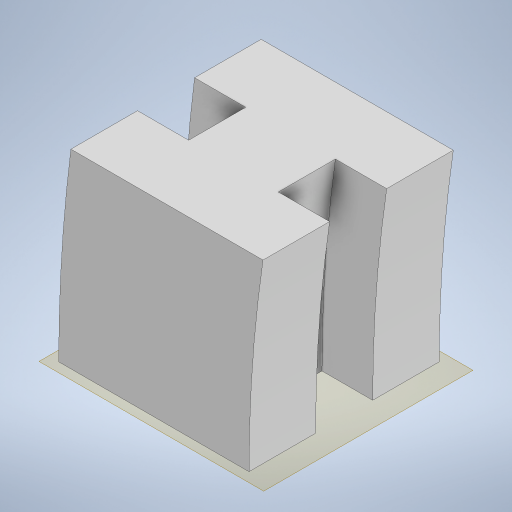
# Autodesk Inventor part: LightRail01
Saved by Autodesk Inventor 2023 (Build 270158000, 158)
## iProperties
Created: 2023-04-11
Part Number: LightRail01
Material: Generic
Document SubType Name: Modeling
Designer: ringl
Density: 1 g/cm^3
Appearance: Default
Author: ringl
Autodesk Inventor part; units mm, degrees
ref_plane "YZ Plane" through (0, 0, 0) normal (1, 0, 0) x (0, 1, 0)
ref_plane "XY Plane" through (0, 0, 0) normal (0, 0, 1) x (1, 0, 0)
sketch "Sketch1" plane through (0, 0, 0) normal (0, 0, 1) x (1, 0, 0)
  arc A0 (440, 0) -> (0, 0) centre (220, 0) ccw
  dimension "d1" = 440
  dimension "d17" = 220
  constraints: 2 point on circle, 1 centre point, 1 horizontal alignment
  measures "d1" distance of A0.end A0.start
  measures "d17" radius of A0
sketch "Sketch2" plane through (0, 0, 0) normal (0, 1, 0) x (-1, 0, 0)
  line L0 (15, 15) -> (-15, 15)
  line L1 (-15, -15) -> (15, -15)
  line L2 (15, 4.5) -> (7, 4.5)
  line L3 (7, 4.5) -> (7, -4.5)
  line L4 (7, -4.5) -> (15, -4.5)
  line L5 (-15, 4.5) -> (-7, 4.5)
  line L6 (-7, 4.5) -> (-7, -4.5)
  line L7 (-7, -4.5) -> (-15, -4.5)
  line L8 (15, -15) -> (15, -4.5)
  line L9 (15, 4.5) -> (15, 15)
  line L10 (-15, 15) -> (-15, 4.5)
  line L11 (-15, -4.5) -> (-15, -15)
  point P0 (0, 0)
  dimension "d18" = 9
  dimension "d19" = 8
  dimension "d21" = 14
  dimension "d22" = 30
  dimension "d23" = 15
  dimension "d24" = 4.5
  dimension "d25" = 7
  constraints: 24 end point, 7 parallel, 4 perpendicular, 3 equal length, 3 horizontal, 2 point on line
  measures "d18" distance of L5.end L6.end
  measures "d19" distance of L5.start L5.end
  measures "d21" distance between parallel lines of L3 L6
  measures "d22" distance between parallel lines of L1 L0
  measures "d23" distance from line of L1 point (0, 0)
  measures "d24" distance from line of point (0, 0) L5
  measures "d25" distance from line of L6 point (0, 0)
sweep "Sweep1" add profiles "Sketch2" path "Sketch1"
sketch "Sketch4" plane through (-15, 0, 15) normal (0, 0, 1) x (1, 0, 0)
  line L0 (470, 0) -> (440, 0) projected
  line L1 (470, 0) -> (51.3779, 0)
  line L2 (51.3779, 0) -> (51.3779, 30)
  line L3 (51.3779, 30) -> (0.5743, 30)
  line L4 (0.5743, 30) -> (0.5743, 269.0711)
  line L5 (0.5743, 269.0711) -> (470, 269.0711)
  line L6 (470, 269.0711) -> (470, 0)
  point P0 (15, 0)
  dimension "d34" = 469.4257
  dimension "d35" = 30
  dimension "d36" = 50.8036
  dimension "d37" = 269.0711
  constraints: 12 end point, 5 perpendicular, 1 horizontal
  measures "d34" distance of L4.end L5.end
  measures "d35" distance of L1.end L2.end
  measures "d36" distance of L2.end L3.end
  measures "d37" distance of L5.end L0.start
extrude "Extrusion2" cut sketch "Sketch4" against normal through all
body "Solid1"
